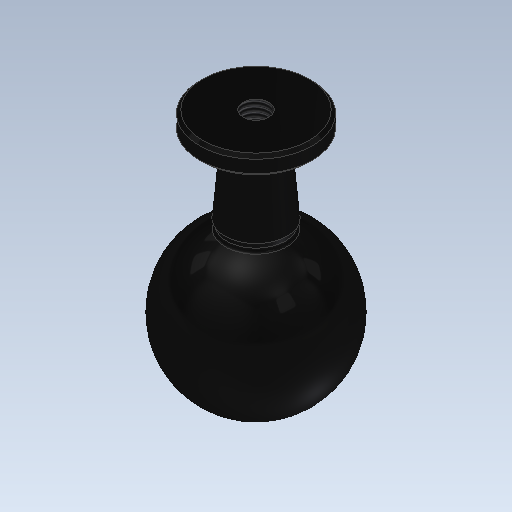
# Autodesk Inventor part: Ball Joint
Saved by Autodesk Inventor 2020 (Build 240168000, 168)
## iProperties
Created: 2012-10-13
Part Number: Ball Joint
Material: Steel, Mild
Document SubType Name: Modeling
Designer: Lance
Mass: 75.5911 g
Surface Area: 30.0384 cm^2
Volume: 9.62943 cm^3
Density: 7.85 g/cm^3
Appearance: Glossy - Black
Author: Lance
Autodesk Inventor part; units mm, degrees
ref_plane "YZ Plane" through (0, 0, 0) normal (1, 0, 0) x (0, 1, 0)
ref_plane "XZ Plane" through (0, 0, 0) normal (0, 1, 0) x (-1, 0, 0)
ref_plane "XY Plane" through (0, 0, 0) normal (0, 0, 1) x (1, 0, 0)
sketch "Sketch1" plane through (0, 0, 0) normal (0, 0, 1) x (1, 0, 0)
  arc A0 (0, 12.5) -> (0, -12.5) centre (0, 0) ccw
  line L0 (0, -17.5) -> (0, 17.5) projected
  dimension "d0" = 25
  constraints: 2 point on circle, 2 point on line, 1 centre point, 1 coincident
  measures "d0" diameter of A0
revolve "Revolution1" add sketch "Sketch1" angle 360 about axis through (0, -10, 0) along (0, 1, 0)
sketch "Sketch2" plane through (0, 0, 0) normal (0, 0, 1) x (1, 0, 0)
  circle A0 centre (0, 0) radius 12.5 projected
  line L0 (0, 0) -> (5, 13)
  line L1 (5, 13) -> (4, 25)
  line L2 (4, 25) -> (9, 25)
  line L3 (9, 25) -> (9, 28)
  line L4 (9, 28) -> (0, 28)
  line L5 (0, -22.3842) -> (0, 46.8051) projected
  line L6 (0, 28) -> (0, 0)
  dimension "d2" = 3
  dimension "d3" = 18
  dimension "d4" = 10
  dimension "d5" = 8
  dimension "d6" = 25
  dimension "d7" = 13
  constraints: 12 end point, 1 collinear, 1 parallel, 1 perpendicular, 1 point on line, 1 vertical
  measures "d2" distance between parallel lines of L2 L4
  measures "d3" diameter of L3 L5
  measures "d4" diameter of L0.end L5
  measures "d5" diameter of L1.end L5
  measures "d6" distance from line of point (0, 0) L2
  measures "d7" vertical distance of L0.end point (0, 0)
revolve "Revolution2" add sketch "Sketch2" angle 360 about axis through (0, -10, 0) along (0, 1, 0) picked at (0.5087, 8.3022) contours L0 L5 A0 | A0 L5 L4 L3 L2 L1 L0
hole "Hole1" at (0, 28, 0) direction (0, -1, 0) diameter 4.134 depth 12 tip angle 118 thread size "M5x0.8" class "6H" standard "ISO Metric profile"
fillet "Fillet1" radius 2 1 edges at (-4, 25, 0)
chamfer "Chamfer1" distance 0.5 angle 45 2 edges at (-9, 25, 0) (-9, 28, 0)
fillet "Fillet2" radius 0.5 2 edges at (0, 11.6668, 4.4872) (0.0001, 11.6668, -4.4872)
body "Solid1"
